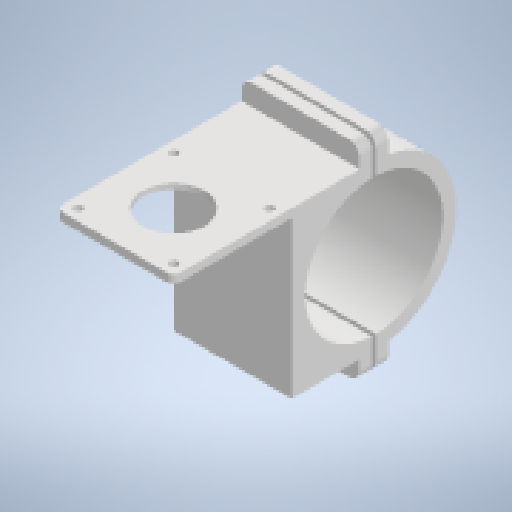
# Autodesk Inventor part: mocowanie_silnika_członu_3
Saved by Autodesk Inventor 2023 (Build 270158000, 158)
## iProperties
Created: 2023-04-24
Part Number: mocowanie_silnika_członu_3
Material: Ogólny
Document SubType Name: Modeling
Designer: krzys
Density: 1 g/cm^3
Appearance: Domyślna
Author: krzys
Autodesk Inventor part; units mm, degrees
ref_plane "YZ Plane" through (0, 0, 0) normal (1, 0, 0) x (0, 1, 0)
ref_plane "XZ Plane" through (0, 0, 0) normal (0, 1, 0) x (-1, 0, 0)
ref_plane "XY Plane" through (0, 0, 0) normal (0, 0, 1) x (1, 0, 0)
sketch "Szkic1" plane through (0, 0, 0) normal (0, 1, 0) x (-1, 0, 0)
  line L0 (5, 272.4746) -> (81, 272.4746)
  line L1 (86, 267.4746) -> (86, 186.4746)
  line L2 (86, 186.4746) -> (0, 186.4746)
  line L3 (0, 186.4746) -> (0, 267.4746)
  line L4 (0, 186.4746) -> (0, 180.4746)
  line L5 (0, 180.4746) -> (86, 180.4746)
  line L6 (86, 180.4746) -> (86, 186.4746)
  line L7 (0, 180.4746) -> (0, 66.4746)
  line L8 (0, 66.4746) -> (86, 66.4746)
  line L9 (86, 66.4746) -> (86, 180.4746)
  circle A0 centre (43, 229.4746) radius 30
  line L10 (77.8, 264.2746) -> (8.2, 194.6746) construction
  line L11 (8.2, 264.2746) -> (77.8, 194.6746) construction
  circle A1 centre (77.8, 264.2746) radius 3.25
  circle A2 centre (8.2, 264.2746) radius 3.25
  circle A3 centre (8.2, 194.6746) radius 3.25
  circle A4 centre (77.8, 194.6746) radius 3.25
  circle A5 centre (43, 229.4746) radius 22.5
  arc A6 (5, 272.4746) -> (0, 267.4746) centre (5, 267.4746) ccw
  arc A7 (86, 267.4746) -> (81, 272.4746) centre (81, 267.4746) ccw
  point P0 (0, 0)
  point P1 (0, 272.4746)
  point P2 (86, 272.4746)
  dimension "d0" = 86
  dimension "d1" = 86
  dimension "d2" = 6
  dimension "d3" = 114
  dimension "d4" = 86
  dimension "d22" = 60
  dimension "d23" = 69.6
  dimension "d24" = 69.6
  dimension "d25" = 6.5
  dimension "d26" = 6.5
  dimension "d27" = 6.5
  dimension "d28" = 6.5
  dimension "d29" = 45
  dimension "d32" = 5
  constraints: 24 end point, 8 centre point, 6 point on line, 5 coincident, 4 perpendicular, 4 point on circle, 4 tangent, 2 midpoint, 2 parallel, 1 equal radius, 1 horizontal, 1 vertical
  measures "d0" distance of L1.end L2.end
  measures "d1" distance of point (86, 272.475) L1.end
  measures "d2" distance of L2.end L4.end
  measures "d3" distance of L4.end L7.end
  measures "d4" distance of L7.end L8.end
  measures "d22" diameter of A0
  measures "d23" distance of L11.end L10.end
  measures "d24" distance of L10.end L11.start
  measures "d25" diameter of A1
  measures "d26" diameter of A2
  measures "d27" diameter of A3
  measures "d28" diameter of A4
  measures "d29" diameter of A5
  measures "d32" radius of A6
extrude "Wyciągnięcie proste1" add sketch "Szkic1" against normal blind 6 contours L0 A7 L1 L2 L3 A6
extrude "Wyciągnięcie proste2" add sketch "Szkic1" against normal blind 120 contours L2 L6 L5 L4
extrude "Wyciągnięcie proste3" add sketch "Szkic1" against normal blind 120 contours L5 L9 L8 L7
sketch "Szkic3" plane through (0, -120, 186.4746) normal (1, 0, 0) x (0, 0, -1)
  line L0 (49.5, 135) -> (70.5, 135)
  line L1 (49.5, 135) -> (70.5, -15) construction
  line L2 (70.5, 135) -> (49.5, -15) construction
  line L3 (0, 0) -> (120, 0) projected
  line L4 (120, 120) -> (120, 0)
  line L5 (120, 0) -> (0, 0)
  line L6 (0, 0) -> (0, 120)
  line L7 (0, 120) -> (120, 0) construction
  line L8 (120, 120) -> (0, 0) construction
  line L9 (49.5, -15) -> (49.5, 0)
  line L10 (49.5, 120) -> (49.5, 135)
  line L11 (70.5, 135) -> (70.5, 119.0741)
  line L12 (70.5, 0.9259) -> (70.5, -15)
  arc A0 (70.5, 0.9259) -> (70.5, 119.0741) centre (60, 60) ccw
  line L13 (58.5, 135) -> (61.5, 135)
  line L14 (61.5, -15) -> (58.5, 135) construction
  line L15 (58.5, -15) -> (61.5, 135) construction
  line L16 (70.5, -15) -> (61.5, -15)
  line L17 (58.5, -15) -> (49.5, -15)
  line L18 (58.5, -15) -> (58.5, 10.0225)
  line L19 (61.5, 10.0225) -> (61.5, -15)
  line L20 (61.5, 135) -> (61.5, 109.9775)
  line L21 (58.5, 109.9775) -> (58.5, 135)
  arc A1 (61.5, 10.0225) -> (61.5, 109.9775) centre (60, 60) ccw
  arc A2 (58.5, 109.9775) -> (58.5, 10.0225) centre (60, 60) ccw
  line L22 (0, 120) -> (58.5, 120)
  line L23 (61.5, 120) -> (120, 120)
  line L24 (58.5, -15) -> (61.5, -15)
  point P0 (186.4746, 120)
  point P1 (70.5, 0)
  point P2 (61.5, 0)
  point P3 (58.5, 0)
  point P4 (49.5, 0)
  point P5 (70.5, 120)
  point P6 (120, 60)
  constraints: 48 end point, 13 parallel, 6 midpoint, 6 point on circle, 4 horizontal, 4 perpendicular, 4 point on line, 3 centre point, 1 coincident
extrude "Wyciągnięcie proste4" add sketch "Szkic3" against normal blind 86 contours L0 L21 L22 L10 | L0 L11 L23 L20 | L3 L18 L17 L9 | L3 L12 L16 L19
extrude "Wyciągnięcie proste5" cut sketch "Szkic3" against normal blind 86 contours L0 L20 A1 L19 L3 L18 A2 L21 | L23 L4 A0 L11 | L3 L19 L24 L18 | L4 L3 L12 A0
fillet "Zaokrąglenie1" radius 8 8 edges at (-86, 15, 120.4746) (-86, 15, 132.4746) (0, 15, 120.4746) (0, 15, 132.4746) (-86, -135, 120.4746) (-86, -135, 132.4746) (0, -135, 120.4746) (0, -135, 132.4746)
extrude "Wyciągnięcie proste6" add sketch "Szkic1" against normal blind 4 contours A0
